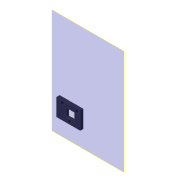
# Autodesk Inventor part: cellSTORM_v5_chiptray_old_0
Saved by Autodesk Inventor 2019.4 (Build 234330000, 330)
## iProperties
Created: 2020-05-10
Part Number: cellSTORM_v5_chiptray_old_0
Material: Generic
Document SubType Name: Modeling
Designer: diederichbenedict
Density: 1 g/cm^3
Appearance: Default
Author: diederichbenedict
Autodesk Inventor part; units mm, degrees
ref_plane "YZ Plane" through (0, 0, 0) normal (1, 0, 0) x (0, 1, 0)
ref_plane "XZ Plane" through (0, 0, 0) normal (0, 1, 0) x (-1, 0, 0)
ref_plane "XY Plane" through (0, 0, 0) normal (0, 0, 1) x (1, 0, 0)
ref_plane "Work Plane1" through (52.5141, 202.7033, 6.4479) normal (0, 0, -1) x (0, 1, 0)
sketch "Sketch1" plane through (52.5141, 202.7033, 6.4479) normal (0, 0, -1) x (0, 1, 0)
  circle A0 centre (-59.8114, -30.5) radius 1.4 construction
  circle A1 centre (-38.8114, -18.3756) radius 1.4 projected
  circle A2 centre (-38.8114, -42.6244) radius 1.4 construction
  circle A3 centre (41, 0) radius 1.65 projected
  circle A4 centre (-9, 0) radius 1.65 projected
  circle A5 centre (-9, 50) radius 1.65 projected
  circle A6 centre (41, 50) radius 1.65 projected
  circle A7 centre (16, 50) radius 1.65 projected
  circle A8 centre (-9, 25) radius 1.65 projected
  circle A9 centre (16, 0) radius 1.65 projected
  circle A10 centre (41, 25) radius 1.65 projected
  line L0 (80, 55) -> (-80, 55) projected
  line L1 (-80, 55) -> (-80, -55) projected
  line L2 (-80, -55) -> (80, -55) projected
  line L3 (80, -55) -> (80, 55) projected
  line L4 (-36.5, 0) -> (-36.5, -50) projected
  line L5 (-14, 0) -> (-36.5, 0) projected
  line L6 (-14, -5) -> (-14, 0) projected
  line L7 (72, -5) -> (-14, -5) projected
  line L8 (72, -50) -> (72, -5) projected
  line L9 (-36.5, -50) -> (72, -50) projected
  line L10 (-4, 45) -> (-4, 5) projected
  line L11 (36, 45) -> (-4, 45) projected
  line L12 (36, 5) -> (36, 45) projected
  line L13 (-4, 5) -> (36, 5) projected
  line L14 (-64.5989, -17.0433) -> (-64.5989, -57.0433) construction
  line L15 (-64.5989, -57.0433) -> (-34.5989, -57.0433) construction
  line L16 (-34.5989, -57.0433) -> (-34.5989, -17.0433) construction
  line L17 (-34.5989, -17.0433) -> (-64.5989, -17.0433) construction
  line L18 (-34.8114, -13.0433) -> (-63.8114, -13.0433)
  line L19 (-63.8114, -13.0433) -> (-63.8114, -52.6244)
  line L20 (-63.8114, -52.6244) -> (-34.8114, -52.6244)
  line L21 (-34.8114, -52.6244) -> (-34.8114, -13.0433)
  circle A11 centre (-59.8114, -30.5) radius 2.95
  circle A12 centre (-38.8114, -18.3756) radius 2.95
  circle A13 centre (-38.8114, -42.6244) radius 2.95 construction
  line L22 (-36.5, -35.1157) -> (-41.75, -35.1157) construction
  line L23 (-41.75, -35.1157) -> (-41.75, -38.5657) construction
  line L24 (-41.75, -38.5657) -> (-56.86, -38.5657) construction
  line L25 (-56.86, -38.5657) -> (-56.86, -35.1157) construction
  line L26 (-56.86, -35.1157) -> (-60.26, -35.1157) construction
  line L27 (-60.26, -35.1157) -> (-60.26, -52.0657) construction
  line L28 (-60.26, -52.0657) -> (-36.5, -52.0657) construction
  line L29 (-36.5, -52.0657) -> (-36.5, -35.1157) construction
  line L30 (-41.75, -28.3657) -> (-36.5, -28.3657) construction
  line L31 (-36.5, -28.3657) -> (-36.5, -25.0657) construction
  line L32 (-36.5, -25.0657) -> (-60.26, -25.0657) construction
  line L33 (-60.26, -25.0657) -> (-60.26, -28.3657) construction
  line L34 (-60.26, -28.3657) -> (-56.86, -28.3657) construction
  line L35 (-56.86, -28.3657) -> (-56.86, -27.0942) construction
  line L36 (-56.86, -27.0942) -> (-41.75, -27.0942) construction
  line L37 (-41.75, -27.0942) -> (-41.75, -28.3657) construction
  line L38 (-56.86, -35.1157) -> (-60.26, -35.1157) construction
  line L39 (-56.86, -38.5657) -> (-56.86, -35.1157) construction
  line L40 (-41.75, -38.5657) -> (-56.86, -38.5657) construction
  line L41 (-41.75, -35.1157) -> (-41.75, -38.5657) construction
  line L42 (-36.5, -35.1157) -> (-41.75, -35.1157) construction
  line L43 (-36.5, -35.05) -> (-36.5, -35.1157) construction
  line L44 (-36.5, -35.05) -> (-56.86, -35.05) construction
  line L45 (-36.5, -34.78) -> (-36.5, -35.05) construction
  line L46 (-36.5, -34.78) -> (-56.86, -34.78) construction
  line L47 (-36.5, -34.51) -> (-36.5, -34.78) construction
  line L48 (-36.5, -34.51) -> (-56.86, -34.51) construction
  line L49 (-36.5, -34.24) -> (-36.5, -34.51) construction
  line L50 (-36.5, -34.24) -> (-56.86, -34.24) construction
  line L51 (-36.5, -33.97) -> (-36.5, -34.24) construction
  line L52 (-36.5, -33.97) -> (-56.86, -33.97) construction
  line L53 (-36.5, -33.7) -> (-36.5, -33.97) construction
  line L54 (-36.5, -33.7) -> (-56.86, -33.7) construction
  line L55 (-36.5, -33.43) -> (-36.5, -33.7) construction
  line L56 (-36.5, -33.43) -> (-56.86, -33.43) construction
  line L57 (-36.5, -33.16) -> (-36.5, -33.43) construction
  line L58 (-36.5, -33.16) -> (-56.86, -33.16) construction
  line L59 (-36.5, -32.89) -> (-36.5, -33.16) construction
  line L60 (-36.5, -32.89) -> (-56.86, -32.89) construction
  line L61 (-36.5, -32.62) -> (-36.5, -32.89) construction
  line L62 (-36.5, -32.62) -> (-56.86, -32.62) construction
  line L63 (-36.5, -32.35) -> (-36.5, -32.62) construction
  line L64 (-36.5, -32.35) -> (-56.86, -32.35) construction
  line L65 (-36.5, -32.08) -> (-36.5, -32.35) construction
  line L66 (-36.5, -32.08) -> (-56.86, -32.08) construction
  line L67 (-36.5, -31.81) -> (-36.5, -32.08) construction
  line L68 (-36.5, -31.81) -> (-56.86, -31.81) construction
  line L69 (-36.5, -31.54) -> (-36.5, -31.81) construction
  line L70 (-36.5, -31.54) -> (-56.86, -31.54) construction
  line L71 (-36.5, -31.27) -> (-36.5, -31.54) construction
  line L72 (-36.5, -31.27) -> (-56.86, -31.27) construction
  line L73 (-36.5, -31) -> (-36.5, -31.27) construction
  line L74 (-36.5, -31) -> (-56.86, -31) construction
  line L75 (-36.5, -30.73) -> (-36.5, -31) construction
  line L76 (-36.5, -30.73) -> (-56.86, -30.73) construction
  line L77 (-36.5, -30.46) -> (-36.5, -30.73) construction
  line L78 (-36.5, -30.46) -> (-56.86, -30.46) construction
  line L79 (-36.5, -30.19) -> (-36.5, -30.46) construction
  line L80 (-36.5, -30.19) -> (-56.86, -30.19) construction
  line L81 (-36.5, -29.92) -> (-36.5, -30.19) construction
  line L82 (-36.5, -29.92) -> (-56.86, -29.92) construction
  line L83 (-36.5, -29.65) -> (-36.5, -29.92) construction
  line L84 (-36.5, -29.65) -> (-56.86, -29.65) construction
  line L85 (-36.5, -29.38) -> (-36.5, -29.65) construction
  line L86 (-36.5, -29.38) -> (-56.86, -29.38) construction
  line L87 (-36.5, -29.11) -> (-36.5, -29.38) construction
  line L88 (-36.5, -29.11) -> (-56.86, -29.11) construction
  line L89 (-36.5, -28.84) -> (-36.5, -29.11) construction
  line L90 (-36.5, -28.84) -> (-56.86, -28.84) construction
  line L91 (-36.5, -28.3657) -> (-36.5, -28.84) construction
  line L92 (-41.75, -28.3657) -> (-36.5, -28.3657) construction
  line L93 (-41.75, -27.0942) -> (-41.75, -28.3657) construction
  line L94 (-56.86, -27.0942) -> (-41.75, -27.0942) construction
  line L95 (-56.86, -28.3657) -> (-56.86, -27.0942) construction
  line L96 (-60.26, -28.3657) -> (-56.86, -28.3657) construction
  line L97 (-60.26, -35.1157) -> (-60.26, -28.3657) construction
  line L98 (-60.26, -25.0657) -> (-36.5, -25.0657) construction
  line L99 (-36.5, -25.0657) -> (-36.5, -52.0657) construction
  line L100 (-60.26, -52.0657) -> (-60.26, -25.0657) construction
  line L101 (-57.1632, -22.5233) -> (-33.4032, -22.5233) construction
  line L102 (-33.4032, -22.5233) -> (-33.4032, -49.5233) construction
  line L103 (-33.4032, -49.5233) -> (-57.1632, -49.5233) construction
  line L104 (-57.1632, -49.5233) -> (-57.1632, -22.5233) construction
  circle A14 centre (-38.8114, -42.6244) radius 2.95
  point P0 (-202.7033, -52.5141)
  point P1 (-56.7146, -27.9576)
  dimension "d0" = 4
  dimension "d2" = 4
  dimension "d3" = 4
  dimension "d4" = 5.9
  dimension "d5" = 5.9
  dimension "d6" = 5.9
  dimension "d10" = 10
  constraints: 22 end point, 5 parallel, 4 centre point, 4 coincident, 3 horizontal, 3 perpendicular, 1 concentric, 1 other
  measures "d0" distance between parallel lines of L18 L17
  measures "d2" distance from line of L21 A1.centre
  measures "d3" distance from line of L19 A0.centre
  measures "d4" diameter of A11
  measures "d5" diameter of A12
  measures "d6" diameter of A13
  measures "d10" distance from line of L20 A2.centre
extrude "Extrusion1" add sketch "Sketch1" along normal blind 2.5 contours L18 L21 L9 L4 A14 A12 | L4 A12 A14 L9 L21 L20 L19 L18
sketch "Sketch2" plane through (52.5141, 202.7033, 3.9479) normal (0, 0, -1) x (-1, 0, 0)
  circle A0 centre (42.6244, -38.8114) radius 2.95 projected
  circle A1 centre (18.3756, -38.8114) radius 2.95 projected
  circle A2 centre (30.5, -59.8114) radius 2.95 projected
  line L0 (13.0433, -34.8114) -> (13.0433, -63.8114) projected
  line L1 (13.0433, -63.8114) -> (52.6244, -63.8114) projected
  line L2 (52.6244, -63.8114) -> (52.6244, -34.8114) projected
  line L3 (52.6244, -34.8114) -> (13.0433, -34.8114) projected
  point P0 (52.5141, -202.7033)
extrude "Extrusion2" add sketch "Sketch2" along normal blind 2.5 contours A0 | A1 | A2 | L3 L2 L1 L0
sketch "Sketch6" plane through (52.5141, 202.7033, 1.4479) normal (0, 0, -1) x (-1, 0, 0)
  line L0 (13.0433, -34.8114) -> (13.0433, -63.8114) projected
  line L1 (13.0433, -63.8114) -> (52.6244, -63.8114) projected
  line L2 (52.6244, -63.8114) -> (52.6244, -34.8114) projected
  line L3 (52.6244, -34.8114) -> (13.0433, -34.8114) projected
  line L4 (36.772, -42.2392) -> (22.772, -42.2392)
  line L5 (22.772, -42.2392) -> (22.772, -56.2392)
  line L6 (22.772, -56.2392) -> (36.772, -56.2392)
  line L7 (36.772, -56.2392) -> (36.772, -42.2392)
  point P0 (52.5141, -202.7033)
  dimension "d33" = 14
  dimension "d34" = 14
  constraints: 8 end point, 2 parallel, 1 horizontal, 1 perpendicular
  measures "d33" distance of L6.end L5.end
  measures "d34" distance of L5.end L4.end
extrude "Extrusion6" cut sketch "Sketch6" against normal through all contours L7 L6 L5 L4
sketch "Sketch7" plane through (52.5141, 202.7033, 1.4479) normal (0, 0, -1) x (-1, 0, 0)
  line L0 (22.772, -56.2392) -> (22.772, -42.2392) projected
  line L1 (22.772, -42.2392) -> (36.772, -42.2392) projected
  line L2 (36.772, -42.2392) -> (36.772, -56.2392) projected
  line L3 (36.772, -56.2392) -> (22.772, -56.2392) projected
  line L4 (13.0433, -34.8114) -> (13.0433, -63.8114) projected
  line L5 (13.0433, -63.8114) -> (52.6244, -63.8114) projected
  line L6 (52.6244, -63.8114) -> (52.6244, -34.8114) projected
  line L7 (52.6244, -34.8114) -> (13.0433, -34.8114) projected
  line L8 (39.772, -59.2392) -> (39.772, -39.2392)
  line L9 (39.772, -39.2392) -> (19.772, -39.2392)
  line L10 (19.772, -39.2392) -> (19.772, -59.2392)
  line L11 (19.772, -59.2392) -> (39.772, -59.2392)
  point P0 (52.5141, -202.7033)
  dimension "d37" = 20
  constraints: 8 end point, 3 other
  measures "d37" distance between parallel lines of L11 L9
extrude "Extrusion7" cut sketch "Sketch7" against normal blind 0.5 contours L11 L10 L9 L8
sketch "Sketch8" plane through (52.5141, 202.7033, 1.4479) normal (0, 0, -1) x (-1, 0, 0)
  line L0 (19.772, -39.2392) -> (39.772, -39.2392) projected
  line L1 (39.772, -39.2392) -> (39.772, -59.2392) projected
  line L2 (39.772, -59.2392) -> (19.772, -59.2392) projected
  line L3 (19.772, -59.2392) -> (19.772, -39.2392) projected
  line L4 (13.0433, -34.8114) -> (13.0433, -63.8114) projected
  line L5 (13.0433, -63.8114) -> (52.6244, -63.8114) projected
  line L6 (52.6244, -63.8114) -> (52.6244, -34.8114) projected
  line L7 (52.6244, -34.8114) -> (13.0433, -34.8114) projected
  line L8 (41.772, -61.2392) -> (41.772, -37.2392)
  line L9 (41.772, -37.2392) -> (17.772, -37.2392)
  line L10 (17.772, -37.2392) -> (17.772, -61.2392)
  line L11 (17.772, -61.2392) -> (41.772, -61.2392)
  point P0 (52.5141, -202.7033)
  dimension "d40" = 2
  constraints: 8 end point, 3 other
  measures "d40" distance between parallel lines of L1 L8
extrude "Extrusion8" add sketch "Sketch8" along normal blind 1.5 contours L11 L10 L9 L8
sketch "Sketch9" plane through (-0.1103, 138.8919, 6.4479) normal (0, -1, 0) x (1, 0, 0)
  line L0 (12.8524, -4.5) -> (32.8524, -4.5) projected
  line L1 (34.8524, -6.5) -> (10.8524, -6.5) projected
  arc A0 (18.6327, -4.7963) -> (17.8272, -4.7963) centre (18.2299, -4.5) ccw
  line L2 (18.6327, -4.7963) -> (17.8272, -4.7963)
  line L3 (17.8272, -4.7963) -> (17.8272, -6.9787)
  line L4 (17.8272, -6.9787) -> (18.6327, -6.9787)
  line L5 (18.6327, -6.9787) -> (18.6327, -4.7963)
  point P0 (0.1103, -6.4479)
  dimension "d43" = 1
  constraints: 8 end point, 2 parallel, 2 point on circle, 1 centre point, 1 horizontal, 1 perpendicular
  measures "d43" diameter of A0
extrude "Extrusion9" cut sketch "Sketch9" against normal through all
sketch "Sketch10" plane through (52.5141, 202.7033, 6.4479) normal (0, 0, 1) x (1, 0, 0)
  circle A0 centre (-42.6244, -38.8114) radius 2.95 projected
  circle A1 centre (-30.5, -59.8114) radius 2.95 projected
  circle A2 centre (-18.3756, -38.8114) radius 2.95 projected
  point P0 (-52.5141, -202.7033)
extrude "Extrusion10" cut sketch "Sketch10" against normal blind 4
body "Solid1"
